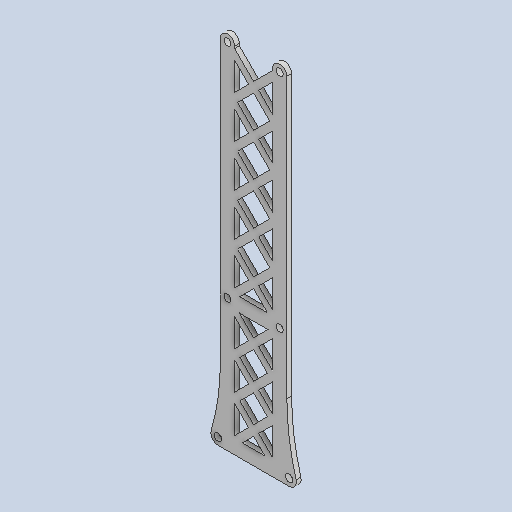
# Autodesk Inventor part: lacznik
Saved by Autodesk Inventor 2023 (Build 270158000, 158)
## iProperties
Created: 2024-04-23
Part Number: lacznik
Material: Ogólny
Document SubType Name: Modeling
Designer: Kamil
Density: 1 g/cm^3
Appearance: Domyślna
Author: Kamil
Autodesk Inventor part; units mm, degrees
ref_plane "YZ Plane" through (0, 0, 0) normal (1, 0, 0) x (0, 1, 0)
ref_plane "XZ Plane" through (0, 0, 0) normal (0, 1, 0) x (-1, 0, 0)
ref_plane "XY Plane" through (0, 0, 0) normal (0, 0, 1) x (1, 0, 0)
sketch "Szkic1" plane through (0, 0, 0) normal (0, 0, 1) x (1, 0, 0)
  circle A0 centre (11, 115) radius 1.55 projected
  circle A1 centre (-11, 115) radius 1.55 projected
  circle A2 centre (11, 21.7) radius 1.55 projected
  circle A3 centre (-11, 21.7) radius 1.55 projected
  line L0 (11, 115) -> (11, 21.7) construction
  line L1 (8, 115) -> (8, 21.7)
  line L2 (14, 21.7) -> (14, 115)
  arc A4 (14, 115) -> (8, 115) centre (11, 115) ccw
  arc A5 (8, 21.7) -> (14, 21.7) centre (11, 21.7) ccw
  line L3 (-11, 115) -> (-11, 21.7) construction
  line L4 (-14, 115) -> (-14, 21.7)
  line L5 (-8, 21.7) -> (-8, 115)
  arc A6 (-8, 115) -> (-14, 115) centre (-11, 115) ccw
  arc A7 (-14, 21.7) -> (-8, 21.7) centre (-11, 21.7) ccw
  line L6 (11, 115) -> (-11, 93)
  line L7 (-11, 21.7) -> (11, 43.7)
  line L8 (-11, 21.7) -> (11, 43.7) construction
  line L9 (-9.9393, 20.6393) -> (12.0607, 42.6393)
  line L10 (9.9393, 44.7607) -> (-12.0607, 22.7607)
  arc A8 (-12.0607, 22.7607) -> (-9.9393, 20.6393) centre (-11, 21.7) ccw
  arc A9 (12.0607, 42.6393) -> (9.9393, 44.7607) centre (11, 43.7) ccw
  line L11 (11, 115) -> (-11, 93) construction
  line L12 (9.9393, 116.0607) -> (-12.0607, 94.0607)
  line L13 (-9.9393, 91.9393) -> (12.0607, 113.9393)
  arc A10 (12.0607, 113.9393) -> (9.9393, 116.0607) centre (11, 115) ccw
  arc A11 (-12.0607, 94.0607) -> (-9.9393, 91.9393) centre (-11, 93) ccw
  line L14 (0, 68.35) -> (-11, 57.35)
  line L15 (0, 68.35) -> (11.1005, 79.4505)
  line L16 (-11, 79.35) -> (11, 57.35)
  line L17 (11, 79.35) -> (-11, 57.35) construction
  line L18 (-11, 79.35) -> (11, 57.35) construction
  line L19 (-11, 115) -> (11, 93) construction
  line L20 (-12.0607, 113.9393) -> (9.9393, 91.9393)
  line L21 (12.0607, 94.0607) -> (-9.9393, 116.0607)
  arc A12 (-9.9393, 116.0607) -> (-12.0607, 113.9393) centre (-11, 115) ccw
  arc A13 (9.9393, 91.9393) -> (12.0607, 94.0607) centre (11, 93) ccw
  line L22 (11, 21.7) -> (-11, 43.7) construction
  line L23 (12.0607, 22.7607) -> (-9.9393, 44.7607)
  line L24 (-12.0607, 42.6393) -> (9.9393, 20.6393)
  arc A14 (9.9393, 20.6393) -> (12.0607, 22.7607) centre (11, 21.7) ccw
  arc A15 (-9.9393, 44.7607) -> (-12.0607, 42.6393) centre (-11, 43.7) ccw
  line L25 (11, 79.35) -> (-11, 57.35) construction
  line L26 (9.9393, 80.4107) -> (-12.0607, 58.4107)
  line L27 (-9.9393, 56.2893) -> (12.0607, 78.2893)
  arc A16 (12.0607, 78.2893) -> (9.9393, 80.4107) centre (11, 79.35) ccw
  arc A17 (-12.0607, 58.4107) -> (-9.9393, 56.2893) centre (-11, 57.35) ccw
  line L28 (-11, 79.35) -> (11, 57.35) construction
  line L29 (-12.0607, 78.2893) -> (9.9393, 56.2893)
  line L30 (12.0607, 58.4107) -> (-9.9393, 80.4107)
  arc A18 (-9.9393, 80.4107) -> (-12.0607, 78.2893) centre (-11, 79.35) ccw
  arc A19 (9.9393, 56.2893) -> (12.0607, 58.4107) centre (11, 57.35) ccw
  point P0 (0, 0)
  point P1 (11, 68.35)
  point P2 (-11, 68.35)
  point P3 (0, 32.7)
  point P4 (0, 104)
  point P5 (0, 104)
  point P6 (0, 32.7)
  point P7 (0, 68.35)
  point P8 (0, 68.35)
  point P9 (-8, 93.8787)
  point P10 (-8, 98.1213)
  point P11 (8, 42.8213)
  point P12 (8, 38.5787)
  point P13 (-8, 26.8213)
  point P14 (8, 109.8787)
  point P15 (-8.8787, 19.5787)
  point P16 (8.8787, 117.1213)
  point P17 (0, 104)
  point P18 (0, 32.7)
  point P19 (0, 68.35)
  point P20 (0, 68.35)
  point P21 (-8, 22.5787)
  point P22 (8, 114.1213)
  point P23 (0, 30.5787)
  point P24 (8, 22.5787)
  point P25 (0, 106.1213)
  point P26 (-8, 114.1213)
  point P27 (8, 98.1213)
  point P28 (2.1213, 104)
  point P29 (-8, 109.8787)
  point P30 (-2.1213, 104)
  point P31 (-2.1213, 68.35)
  point P32 (-8, 62.4713)
  point P33 (-8, 74.2287)
  point P34 (2.1213, 68.35)
  point P35 (8, 74.2287)
  point P36 (8, 62.4713)
  point P37 (0, 34.8213)
  point P38 (-8, 42.8213)
  point P39 (-8, 58.2287)
  point P40 (0, 66.2287)
  point P41 (8, 58.2287)
  point P42 (8, 26.8213)
  point P43 (2.1213, 32.7)
  point P44 (0, 101.8787)
  point P45 (8, 93.8787)
  point P46 (8, 78.4713)
  point P47 (0, 70.4713)
  point P48 (-8, 78.4713)
  point P49 (-8, 38.5787)
  point P50 (-2.1213, 32.7)
  dimension "d1" = 6
  dimension "d2" = 45
  dimension "d3" = 45
  dimension "d4" = 45
  dimension "d5" = 45
  dimension "d8" = 3
  dimension "d9" = 3
  dimension "d10" = 3
  dimension "d11" = 3
  dimension "d13" = 3
  dimension "d14" = 3
  constraints: 82 end point, 32 point on circle, 32 tangent, 16 centre point, 11 midpoint, 11 point on line, 8 parallel, 4 collinear, 2 vertical, 1 other
  measures "d1" diameter of A7
  measures "d2" angle of L1 L6
  measures "d3" angle of L5 L7
  measures "d4" angle of L5 L14
  measures "d5" angle of L1 L16
  measures "d8" distance between parallel lines of L12 L13
  measures "d9" diameter of A13
  measures "d10" distance between parallel lines of L9 L10
  measures "d11" diameter of A15
  measures "d13" diameter of A17
  measures "d14" diameter of A19
extrude "Wyciągnięcie proste2" add sketch "Szkic1" along normal blind 2 contours A0 L13 A10 L12 | A0 L12 L1 A4 L2 A5 L24 A2 L23 L9 A9 L10 L29 A19 L30 L27 A16 L26 L20 A13 L21 L13 | L12 A10 L13 A0 | A0 L6 L1 L12 | L13 L1 L6 A0 | L1 L6 L21 L12 | L13 L21 L6 L1 | L21 L6 L20 L12 | L12 L20 L5 L21 | L21 A13 L20 L1 | L1 L20 L13 L21 | L13 L20 L6 L21 | L20 L6 L5 L12 | L21 A1 L20 L5 L12 A11 L13 L30 A18 L29 L26 A17 L27 L23 A15 L24 L10 A3 L9 A7 L4 A6 | L5 L20 A1 L21 | L13 L5 L6 L20 | L5 L13 A11 L12 | L21 A12 L20 A1 | A1 L20 A12 L21 | L26 A16 L27 L1 | L1 L15 L30 L26 | L1 L27 L30 L15 | L30 L15 L16 L26 | L26 L16 L5 L30 | L5 L29 A18 L30 | L24 L9 L23 L1 | L1 L23 A2 L24 | L30 L27 L16 L15 | L26 L29 L5 L16 | L16 L14 L29 L26 | L24 L7 L23 L9 | L9 L5 L7 L24 | L24 A14 L23 A2 | A2 L23 A14 L24 | L30 A19 L29 L1 | L1 L16 L27 L30 | L16 L27 L29 L14 | L29 L14 L5 L26 | L9 L23 L7 L1 | L1 L10 A9 L9 | L9 A3 L7 L5 | L24 L10 L23 L7 | L7 L5 L10 L24 | L1 L29 L27 L16 | L29 L27 L5 L14 | L5 L27 A17 L26 | L7 L23 L10 L1 | L7 A3 L10 L5 | L9 A8 L10 A3 | A3 L10 A8 L9 | L24 L5 L23 L10 | L24 A15 L23 L5
sketch "Szkic2" plane through (0, 0, 2) normal (0, 0, 1) x (1, 0, 0)
  line L0 (0, 30.5787) -> (8, 22.5787) projected
  line L1 (8, 22.5787) -> (8, 21.7) projected
  arc A0 (8, 21.7) -> (14, 21.7) centre (11, 21.7) ccw projected
  line L2 (14, 21.7) -> (14, 115) projected
  arc A1 (14, 115) -> (8, 115) centre (11, 115) ccw projected
  line L3 (8, 115) -> (8, 114.1213) projected
  line L4 (8, 114.1213) -> (0, 106.1213) projected
  line L5 (0, 106.1213) -> (-8, 114.1213) projected
  line L6 (-8, 114.1213) -> (-8, 115) projected
  arc A2 (-8, 115) -> (-14, 115) centre (-11, 115) ccw projected
  line L7 (-14, 115) -> (-14, 21.7) projected
  arc A3 (-14, 21.7) -> (-8, 21.7) centre (-11, 21.7) ccw projected
  line L8 (-8, 21.7) -> (-8, 22.5787) projected
  line L9 (-8, 22.5787) -> (0, 30.5787) projected
  line L10 (8, 109.8787) -> (8, 98.1213) projected
  line L11 (8, 98.1213) -> (2.1213, 104) projected
  line L12 (2.1213, 104) -> (8, 109.8787) projected
  line L13 (-8, 109.8787) -> (-2.1213, 104) projected
  line L14 (-2.1213, 104) -> (-8, 98.1213) projected
  line L15 (-8, 98.1213) -> (-8, 109.8787) projected
  line L16 (-2.1213, 68.35) -> (-8, 62.4713) projected
  line L17 (-8, 62.4713) -> (-8, 74.2287) projected
  line L18 (-8, 74.2287) -> (-2.1213, 68.35) projected
  line L19 (2.1213, 68.35) -> (8, 74.2287) projected
  line L20 (8, 74.2287) -> (8, 62.4713) projected
  line L21 (8, 62.4713) -> (2.1213, 68.35) projected
  line L22 (0, 34.8213) -> (-8, 42.8213) projected
  line L23 (-8, 42.8213) -> (-8, 58.2287) projected
  line L24 (-8, 58.2287) -> (0, 66.2287) projected
  line L25 (0, 66.2287) -> (8, 58.2287) projected
  line L26 (8, 58.2287) -> (8, 42.8213) projected
  line L27 (8, 42.8213) -> (0, 34.8213) projected
  line L28 (8, 26.8213) -> (2.1213, 32.7) projected
  line L29 (2.1213, 32.7) -> (8, 38.5787) projected
  line L30 (8, 38.5787) -> (8, 26.8213) projected
  line L31 (0, 101.8787) -> (8, 93.8787) projected
  line L32 (8, 93.8787) -> (8, 78.4713) projected
  line L33 (8, 78.4713) -> (0, 70.4713) projected
  line L34 (0, 70.4713) -> (-8, 78.4713) projected
  line L35 (-8, 78.4713) -> (-8, 93.8787) projected
  line L36 (-8, 93.8787) -> (0, 101.8787) projected
  line L37 (-8, 26.8213) -> (-8, 38.5787) projected
  line L38 (-8, 38.5787) -> (-2.1213, 32.7) projected
  line L39 (-2.1213, 32.7) -> (-8, 26.8213) projected
  circle A4 centre (11, 115) radius 1.5
  circle A5 centre (-11, 115) radius 1.5
  circle A6 centre (11, 21.7) radius 1.5
  circle A7 centre (-11, 21.7) radius 1.5
  point P0 (0, 0)
  dimension "d17" = 3
  dimension "d18" = 3
  dimension "d19" = 3
  dimension "d20" = 3
  constraints: 4 centre point, 4 coincident
  measures "d17" diameter of A4
  measures "d18" diameter of A5
  measures "d19" diameter of A6
  measures "d20" diameter of A7
extrude "Wyciągnięcie proste3" cut sketch "Szkic2" against normal blind 2 contours A4 | A5 | A6 | A7
sketch "Szkic3" plane through (0, 0, 0) normal (0, 0, -1) x (-1, 0, 0)
  circle A0 centre (15, -31) radius 1.6 projected
  circle A1 centre (-15, -31) radius 1.6 projected
  circle A2 centre (-11, 21.7) radius 1.5 projected
  circle A3 centre (11, 21.7) radius 1.5 projected
  circle A4 centre (11, 115) radius 1.5 projected
  circle A5 centre (11, 21.7) radius 1.5 projected
  circle A6 centre (-11, 115) radius 1.5 projected
  circle A7 centre (-11, 21.7) radius 1.5 projected
  line L0 (0, 30.5787) -> (-8, 22.5787) projected
  line L1 (8, 22.5787) -> (0, 30.5787) projected
  line L2 (8, 21.7) -> (8, 22.5787) projected
  arc A8 (8, 21.7) -> (14, 21.7) centre (11, 21.7) ccw projected
  line L3 (14, 115) -> (14, 21.7) projected
  arc A9 (14, 115) -> (8, 115) centre (11, 115) ccw projected
  line L4 (8, 114.1213) -> (8, 115) projected
  line L5 (0, 106.1213) -> (8, 114.1213) projected
  line L6 (-8, 114.1213) -> (0, 106.1213) projected
  line L7 (-8, 115) -> (-8, 114.1213) projected
  arc A10 (-8, 115) -> (-14, 115) centre (-11, 115) ccw projected
  line L8 (-14, 21.7) -> (-14, 115) projected
  arc A11 (-14, 21.7) -> (-8, 21.7) centre (-11, 21.7) ccw projected
  line L9 (-8, 22.5787) -> (-8, 21.7) projected
  line L10 (-8, 109.8787) -> (-8, 98.1213) projected
  line L11 (-2.1213, 104) -> (-8, 109.8787) projected
  line L12 (-8, 98.1213) -> (-2.1213, 104) projected
  line L13 (8, 109.8787) -> (2.1213, 104) projected
  line L14 (8, 98.1213) -> (8, 109.8787) projected
  line L15 (2.1213, 104) -> (8, 98.1213) projected
  line L16 (2.1213, 68.35) -> (8, 62.4713) projected
  line L17 (8, 74.2287) -> (2.1213, 68.35) projected
  line L18 (8, 62.4713) -> (8, 74.2287) projected
  line L19 (-2.1213, 68.35) -> (-8, 74.2287) projected
  line L20 (-8, 62.4713) -> (-2.1213, 68.35) projected
  line L21 (-8, 74.2287) -> (-8, 62.4713) projected
  line L22 (0, 34.8213) -> (8, 42.8213) projected
  line L23 (-8, 42.8213) -> (0, 34.8213) projected
  line L24 (-8, 58.2287) -> (-8, 42.8213) projected
  line L25 (0, 66.2287) -> (-8, 58.2287) projected
  line L26 (8, 58.2287) -> (0, 66.2287) projected
  line L27 (8, 42.8213) -> (8, 58.2287) projected
  line L28 (-8, 26.8213) -> (-2.1213, 32.7) projected
  line L29 (-8, 38.5787) -> (-8, 26.8213) projected
  line L30 (-2.1213, 32.7) -> (-8, 38.5787) projected
  line L31 (0, 101.8787) -> (-8, 93.8787) projected
  line L32 (8, 93.8787) -> (0, 101.8787) projected
  line L33 (8, 78.4713) -> (8, 93.8787) projected
  line L34 (0, 70.4713) -> (8, 78.4713) projected
  line L35 (-8, 78.4713) -> (0, 70.4713) projected
  line L36 (-8, 93.8787) -> (-8, 78.4713) projected
  line L37 (8, 26.8213) -> (8, 38.5787) projected
  line L38 (2.1213, 32.7) -> (8, 26.8213) projected
  line L39 (8, 38.5787) -> (2.1213, 32.7) projected
  circle A12 centre (11, 21.7) radius 1.5 projected
  arc A13 (13.9828, 21.9264) -> (8.0172, 21.4736) centre (11, 21.7) ccw
  circle A14 centre (-11, 21.7) radius 1.5 projected
  arc A15 (-8.0172, 21.4736) -> (-13.9828, 21.9264) centre (-11, 21.7) ccw
  line L40 (-11, 21.7) -> (-11, -31) construction
  line L41 (-8, 21.7) -> (-8, -31)
  line L42 (-14, -31) -> (-14, 21.7)
  arc A16 (-8, 21.7) -> (-14, 21.7) centre (-11, 21.7) ccw
  arc A17 (-14, -31) -> (-8, -31) centre (-11, -31) ccw
  line L43 (11, 21.7) -> (11, -31) construction
  line L44 (8.0086, 21.7) -> (8.0086, -31)
  line L45 (13.9914, -31) -> (13.9914, 21.7)
  arc A18 (13.9914, 21.7) -> (8.0086, 21.7) centre (11, 21.7) ccw
  arc A19 (8.0086, -31) -> (13.9914, -31) centre (11, -31) ccw
  line L46 (15, -31) -> (-15, -31) construction
  line L47 (15, -28) -> (-15, -28)
  line L48 (-15, -34) -> (15, -34)
  arc A20 (15, -34) -> (15, -28) centre (15, -31) ccw
  arc A21 (-15, -28) -> (-15, -34) centre (-15, -31) ccw
  point P0 (0, 0)
  point P1 (13, -4.65)
  point P2 (-13, -4.65)
  point P3 (0, -31)
  point P4 (-11, -4.65)
  point P5 (11, -4.65)
  point P6 (0, -31)
  point P7 (13.9914, -28)
  point P8 (13.9914, 21.4729)
  point P9 (8.0086, 21.4729)
  point P10 (8.0086, -28)
  point P11 (-8, -28)
  point P12 (-14, -28)
  constraints: 24 end point, 16 point on circle, 12 tangent, 8 centre point, 4 parallel, 3 midpoint, 2 horizontal alignment, 2 vertical alignment, 1 horizontal, 1 vertical
extrude "Wyciągnięcie proste4" add sketch "Szkic3" against normal up to surface (2 mm away) contours A0 L45 L47 A20 L48 A17 L41 L44 A19 | A0 A19 L44 L47 L45 | L47 L44 A8 L45 | L47 L42 A11 L41 | L41 A17 A1 L42 L47 | L48 A21 L47 L42 A1 A17
sketch "Szkic4" plane through (0, 0, 0) normal (0, 0, -1) x (-1, 0, 0)
  arc A0 (13.9914, 21.4729) -> (14, 21.7) centre (11, 21.7) ccw projected
  line L0 (14, 115) -> (14, 21.7) projected
  arc A1 (14, 115) -> (8, 115) centre (11, 115) ccw projected
  line L1 (8, 114.1213) -> (8, 115) projected
  line L2 (0, 106.1213) -> (8, 114.1213) projected
  line L3 (-8, 114.1213) -> (0, 106.1213) projected
  line L4 (-8, 115) -> (-8, 114.1213) projected
  arc A2 (-8, 115) -> (-14, 115) centre (-11, 115) ccw projected
  line L5 (-14, 115) -> (-14, -28) projected
  line L6 (-14, -28) -> (-15, -28) projected
  arc A3 (-15, -28) -> (-15, -34) centre (-15, -31) ccw projected
  line L7 (-15, -34) -> (15, -34) projected
  arc A4 (15, -34) -> (15, -28) centre (15, -31) ccw projected
  line L8 (15, -28) -> (13.9914, -28) projected
  line L9 (13.9914, -28) -> (13.9914, 21.4729) projected
  circle A5 centre (-15, -31) radius 1.6 projected
  circle A6 centre (15, -31) radius 1.6 projected
  circle A7 centre (11, 115) radius 1.5 projected
  circle A8 centre (11, 21.7) radius 1.5 projected
  circle A9 centre (-11, 115) radius 1.5 projected
  circle A10 centre (-11, 21.7) radius 1.5 projected
  line L10 (8.0086, 21.4729) -> (8.0086, -28) projected
  line L11 (8.0086, -28) -> (-8, -28) projected
  line L12 (-8, 22.5787) -> (-8, -28) projected
  line L13 (0, 30.5787) -> (-8, 22.5787) projected
  line L14 (8, 22.5787) -> (0, 30.5787) projected
  line L15 (8, 21.7) -> (8, 22.5787) projected
  arc A11 (8, 21.7) -> (8.0086, 21.4729) centre (11, 21.7) ccw projected
  line L16 (-8, 109.8787) -> (-8, 98.1213) projected
  line L17 (-2.1213, 104) -> (-8, 109.8787) projected
  line L18 (-8, 98.1213) -> (-2.1213, 104) projected
  line L19 (8, 109.8787) -> (2.1213, 104) projected
  line L20 (8, 98.1213) -> (8, 109.8787) projected
  line L21 (2.1213, 104) -> (8, 98.1213) projected
  line L22 (2.1213, 68.35) -> (8, 62.4713) projected
  line L23 (8, 74.2287) -> (2.1213, 68.35) projected
  line L24 (8, 62.4713) -> (8, 74.2287) projected
  line L25 (-2.1213, 68.35) -> (-8, 74.2287) projected
  line L26 (-8, 62.4713) -> (-2.1213, 68.35) projected
  line L27 (-8, 74.2287) -> (-8, 62.4713) projected
  line L28 (0, 34.8213) -> (8, 42.8213) projected
  line L29 (-8, 42.8213) -> (0, 34.8213) projected
  line L30 (-8, 58.2287) -> (-8, 42.8213) projected
  line L31 (0, 66.2287) -> (-8, 58.2287) projected
  line L32 (8, 58.2287) -> (0, 66.2287) projected
  line L33 (8, 42.8213) -> (8, 58.2287) projected
  line L34 (-8, 26.8213) -> (-2.1213, 32.7) projected
  line L35 (-8, 38.5787) -> (-8, 26.8213) projected
  line L36 (-2.1213, 32.7) -> (-8, 38.5787) projected
  line L37 (0, 101.8787) -> (-8, 93.8787) projected
  line L38 (8, 93.8787) -> (0, 101.8787) projected
  line L39 (8, 78.4713) -> (8, 93.8787) projected
  line L40 (0, 70.4713) -> (8, 78.4713) projected
  line L41 (-8, 78.4713) -> (0, 70.4713) projected
  line L42 (-8, 93.8787) -> (-8, 78.4713) projected
  line L43 (8, 26.8213) -> (8, 38.5787) projected
  line L44 (2.1213, 32.7) -> (8, 26.8213) projected
  line L45 (8, 38.5787) -> (2.1213, 32.7) projected
  line L46 (0, 88.2963) -> (6.7912, 95.0875)
  line L47 (-6.7912, 95.0875) -> (0, 88.2963)
  line L48 (-2.1213, 86.175) -> (-8, 92.0537)
  line L49 (-8, 80.2963) -> (-2.1213, 86.175)
  line L50 (8, 92.0537) -> (2.1213, 86.175)
  line L51 (2.1213, 86.175) -> (8, 80.2963)
  line L52 (0, 84.0537) -> (-6.7912, 77.2625)
  line L53 (6.7912, 77.2625) -> (0, 84.0537)
  line L54 (0, 101.8787) -> (0, 70.4713) construction
  line L55 (0, 66.2287) -> (-8, 58.2287) construction
  line L56 (0, 66.2287) -> (0, 34.8213) construction
  line L57 (0, 30.5787) -> (-8, 22.5787) construction
  line L58 (0, 52.6463) -> (6.7912, 59.4375)
  line L59 (-6.7912, 59.4375) -> (0, 52.6463)
  line L60 (0, 48.4037) -> (-6.7912, 41.6125)
  line L61 (6.7912, 41.6125) -> (0, 48.4037)
  line L62 (-8, 44.6463) -> (-2.1213, 50.525)
  line L63 (2.1213, 50.525) -> (8, 44.6463)
  line L64 (8, 56.4037) -> (2.1213, 50.525)
  line L65 (-2.1213, 50.525) -> (-8, 56.4037)
  line L66 (11, 21.7) -> (-11, 21.7) construction
  line L67 (11, 24.7) -> (-11, 24.7)
  line L68 (-11, 18.7) -> (11, 18.7)
  arc A12 (11, 18.7) -> (11, 24.7) centre (11, 21.7) ccw
  arc A13 (-11, 24.7) -> (-11, 18.7) centre (-11, 21.7) ccw
  line L69 (2.1299, 10.558) -> (8.0086, 4.6793)
  line L70 (8.0086, 16.4367) -> (2.1299, 10.558)
  line L71 (0, 12.6793) -> (6.0207, 18.7)
  line L72 (-8, 4.6793) -> (-2.1213, 10.558)
  line L73 (-6.0207, 18.7) -> (0, 12.6793)
  line L74 (-2.1213, 10.558) -> (-8, 16.4367)
  line L75 (2.1256, -5.2783) -> (8.0086, -11.1613)
  line L76 (8.0086, 0.6047) -> (2.1256, -5.2783)
  line L77 (-8, -11.1527) -> (-2.1213, -5.274)
  line L78 (-2.1213, -5.274) -> (-8, 0.6047)
  line L79 (2.1299, -21.106) -> (8.0086, -26.9847)
  line L80 (8, -31.2273) -> (0, -23.2273)
  line L81 (8.0086, -15.2273) -> (2.1299, -21.106)
  line L82 (0, -23.2273) -> (-8, -31.2273)
  line L83 (-8, -26.9847) -> (-2.1213, -21.106)
  line L84 (-5.7947, -13.19) -> (0, -18.9847)
  line L85 (-2.1213, -21.106) -> (-8, -15.2273)
  line L86 (0, -3.1527) -> (5.7947, 2.642)
  line L87 (5.7947, 2.642) -> (0, 8.4367)
  line L88 (-5.7947, 2.642) -> (0, -3.1527)
  line L89 (0, 8.4367) -> (-5.7947, 2.642)
  line L90 (0, -7.3953) -> (-5.7947, -13.19)
  line L91 (0, -18.9847) -> (5.7947, -13.19)
  line L92 (5.7947, -13.19) -> (0, -7.3953)
  point P0 (0, 0)
  point P1 (0, 86.175)
  point P2 (0, 86.175)
  point P3 (0, 50.525)
  point P4 (0, 50.525)
  point P5 (0, 21.7)
  point P6 (0, 10.558)
  point P7 (0, -5.274)
  point P8 (0, 18.7)
  point P9 (0, 68.6463)
  point P10 (0, 32.8418)
  point P11 (0, -21.106)
  point P12 (0, 10.558)
  point P13 (0, -5.274)
  point P14 (0, -21.106)
  point P15 (5.8787, 24.7)
  point P16 (-5.8787, 24.7)
  point P17 (-4.7727, -28)
  point P18 (4.7727, -28)
  dimension "d29" = 15.832
  dimension "d30" = 11.142
  dimension "d31" = 15.832
  constraints: 92 end point, 16 point on line, 5 tangent, 4 midpoint, 4 point on circle, 3 vertical alignment, 2 centre point, 2 equal length, 1 horizontal
  measures "d29" distance of point (0, 10.558) point (0, -5.274)
  measures "d30" distance of point (0, 10.558) point (0, 21.7)
  measures "d31" distance of point (0, -21.106) point (0, -5.274)
extrude "Wyciągnięcie proste5" add sketch "Szkic4" against normal up to surface (2 mm away) contours L68 L12 L13 L67 L14 L15 A11 L10 | L10 L70 L69 L76 L75 L81 L79 L11 L80 L82 L12 L83 L85 L77 L78 L72 L74 L68 L73 L71 | L61 L60 L29 L30 L62 L65 L31 L59 L58 L32 L33 L64 L63 L28 | L47 L46 L38 L39 L50 L51 L40 L53 L52 L41 L42 L49 L48 L37
fillet "Zaokrąglenie1" radius 100 2 edges at (-13.9914, -28, 1) (14, -28, 1)
